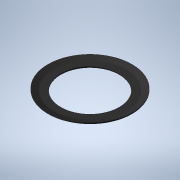
# Autodesk Inventor part: 49200510
Saved by Autodesk Inventor 2021 (Build 250183000, 183)
## iProperties
Created: 2025-04-22
Part Number: 49200510
Material: Generic
Catalog Web Link: www.cadenas.de
Description: Flange 0.5 mm-Zincplated depth 0.5 mm
Vendor: CHIARAVALLI
Document SubType Name: Modeling
Designer: psAdmin
Manufacturer: CHIARAVALLI
Mass: 2 g
Surface Area: 11.6839 cm^2
Volume: 0.263501 cm^3
Density: 1 g/cm^3
Appearance: PSOLRGB-175-175-175
Category: PARTsolutions
Company: CHIARAVALLI
Title: 49200510
Author: Cadenas PARTsolutions
Comments: Zincplated depth 0.5 mm
PSOL_IDENT_0: {$CADENAS_DATA/23d-libs/chiaravalli/open_transmission/flanges_for_pulleys/zincplated_depth_05mm.prj}
PSOL_IDENT_1: ,164 {VTYP=3D},{NB=49200510},{LINA=49200510},{NN=Flange 0.5 mm},{DATE=24.09.2024 10:13:10},{GEOMDATE=
PSOL_IDENT_2: 30.04.2024 13:35:09},{VERSION=},{LINEID=100},{WBVAR=},{WBNUMERIC=}  {NB=49200510},{LINA=49200510},{K
PSOL_IDENT_3: T=DUMMY},{NF=510},{CODE=49200510},{E=36.0},{L=25.0},{M=31.0},{S=0.5},{WEIGHT=0.0020},{MAT=S235 JR EN
PSOL_IDENT_4: 10025}
NB: 49200510
NN: Flange 0.5 mm
NT: Zincplated depth 0.5 mm
NBSYN: $CODE.
LINA: 49200510
CATALOG: Chiaravalli
NF: 510
CODE: 49200510
E: 36
L: 25
M: 31
S: 0.5
WEIGHT: 0.002
MAT: S235 JR EN 10025
SUPPLIER: CHIARAVALLI
ARTICLENO: 49200510
BOMINFO: 49200510
CREATOR: CADENAS GmbH
Autodesk Inventor part; units mm, degrees
sketch "Sketch_1" plane through (0, 0, 0) normal (0, 0, 1) x (1, 0, 0)
  line L0 (0, 0) -> (0, 0.5)
  line L1 (12.5, 0.5) -> (12.5, 0)
  line L2 (12.5, 0) -> (15.5, 0)
  line L3 (15.5, 0) -> (18, 0.6699)
  line L4 (18, 0.6699) -> (18, 1.1699)
  line L5 (18, 1.1699) -> (15.5, 0.5)
  line L6 (15.5, 0.5) -> (12.5, 0.5)
  constraints: 14 end point
revolve "Revolution1" add sketch "Sketch_1" angle 360 about axis through (0, 0, 0) along (0, -1, 0)
ref_plane "FL1_XY" through (0, 0, 0) normal (0, -1, 0) x (1, 0, 0)
ref_plane "FL1_YZ" through (0, 0, 0) normal (1, 0, 0) x (0, 0, 1)
ref_plane "FL1_ZX" through (0, 0, 0) normal (0, 0, 1) x (0, -1, 0)
body "Solid1"
